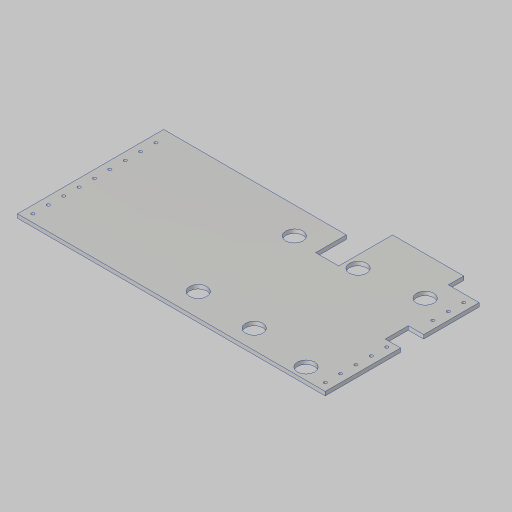
# Autodesk Inventor part: GP3-001
Saved by Autodesk Inventor 2023.5 (Build 275446000, 446)
## iProperties
Created: 2025-02-22
Part Number: GP3-001
Material: Aluminum 6061
Document SubType Name: Modeling
Designer: slick
Density: 2.7 g/cm^3
Appearance: Aluminum - Flat
Author: slick
Autodesk Inventor part; units mm, degrees
ref_plane "YZ Plane" through (0, 0, 0) normal (1, 0, 0) x (0, 1, 0)
ref_plane "XZ Plane" through (0, 0, 0) normal (0, 1, 0) x (-1, 0, 0)
ref_plane "XY Plane" through (0, 0, 0) normal (0, 0, 1) x (1, 0, 0)
sketch "Sketch1" plane through (0, 0, 0) normal (0, 1, 0) x (-1, 0, 0)
  line L0 (-254, -139.7) -> (254, -139.7)
  line L1 (254, -139.7) -> (254, 139.7)
  line L2 (254, 139.7) -> (-254, 139.7)
  line L3 (-254, 139.7) -> (-254, -139.7)
  line L4 (-254, -139.7) -> (254, 139.7) construction
  line L5 (254, -139.7) -> (-254, 139.7) construction
  point P0 (0, 0)
  dimension "d0" = 508
  dimension "d1" = 279.4
  constraints: 12 end point, 2 midpoint, 2 parallel, 1 horizontal, 1 perpendicular
  measures "d0" distance of L2.end L1.end
  measures "d1" distance of L1.end L0.end
extrude "Extrusion1" add sketch "Sketch1" along normal blind 6.35
sketch "Sketch2" plane through (0, 6.35, 0) normal (0, 1, 0) x (1, 0, 0)
  line L0 (-254, 139.7) -> (-254, -139.7) construction
  line L1 (-254, -139.7) -> (254, -139.7) construction
  line L2 (254, -139.7) -> (254, 139.7) construction
  point P0 (0, 0)
  point P1 (-241.3, -127)
  point P2 (241.3, -127)
  point P3 (-241.3, -101.6)
  point P4 (241.3, -101.6)
  point P5 (-241.3, -76.2)
  point P6 (241.3, -76.2)
  point P7 (-241.3, -50.8)
  point P8 (241.3, -50.8)
  point P9 (-241.3, -25.4)
  point P10 (241.3, -25.4)
  point P11 (-241.3, 0)
  point P12 (241.3, 0)
  point P13 (-241.3, 25.4)
  point P14 (241.3, 25.4)
  point P15 (-241.3, 50.8)
  point P16 (241.3, 50.8)
  point P17 (-241.3, 76.2)
  point P18 (241.3, 76.2)
  point P19 (-241.3, 101.6)
  point P20 (241.3, 101.6)
  point P21 (-241.3, 127)
  point P22 (241.3, 127)
  dimension "d4" = 12.7
  dimension "d5" = 12.7
  dimension "d6" = 12.7
  dimension "d9" = 25.4
  constraints: 1 horizontal alignment, 1 vertical, 20 other
  measures "d4" distance from line of point (-241.3, -127) L0
  measures "d5" distance from line of point (-241.3, -127) L1
  measures "d6" distance from line of L2 point (241.3, -127)
  measures "d9" distance of point (-241.3, -127) point (-241.3, -101.6)
hole "Hole1" at (-241.3, 6.35, 127) at (241.3, 6.35, 127) at (-241.3, 6.35, 101.6) at (241.3, 6.35, 101.6) at (-241.3, 6.35, 76.2) at (241.3, 6.35, 76.2) at (-241.3, 6.35, 50.8) at (241.3, 6.35, 50.8) at (-241.3, 6.35, 25.4) at (-241.3, 6.35, 0) at (-241.3, 6.35, -25.4) at (-241.3, 6.35, -50.8) at (241.3, 6.35, -50.8) at (241.3, 6.35, -76.2) at (241.3, 6.35, -101.6) at (241.3, 6.35, -127) at (241.3, 6.35, 25.4) at (-241.3, 6.35, -76.2) direction (0, -1, 0) diameter 5.1054 end through all clearance for "Flat Head Machine Screw (82)" size "#10" standard "Ansi Unified Screw Threads"
sketch "Sketch3" plane through (0, 6.35, 0) normal (0, 1, 0) x (1, 0, 0)
  circle A0 centre (-241.3, 50.8) radius 2.5527 construction
  circle A1 centre (-241.3, 25.4) radius 2.5527 construction
  circle A2 centre (-241.3, 0) radius 2.5527 construction
  circle A3 centre (-241.3, -25.4) radius 2.5527 construction
  circle A4 centre (-241.3, -50.8) radius 2.5527 construction
  circle A5 centre (-241.3, -76.2) radius 2.5527 construction
  circle A6 centre (-241.3, -101.6) radius 2.5527 construction
  circle A7 centre (-241.3, -127) radius 2.5527 construction
  circle A8 centre (241.3, -127) radius 2.5527 construction
  circle A9 centre (241.3, -101.6) radius 2.5527 construction
  circle A10 centre (241.3, -76.2) radius 2.5527 construction
  circle A11 centre (241.3, -50.8) radius 2.5527 construction
  circle A12 centre (241.3, 50.8) radius 2.5527 construction
  circle A13 centre (241.3, 76.2) radius 2.5527 construction
  circle A14 centre (241.3, 101.6) radius 2.5527 construction
  circle A15 centre (241.3, 127) radius 2.5527 construction
  line L0 (-254, 139.7) -> (-254, -139.7) construction
  line L1 (-254, -139.7) -> (254, -139.7) construction
  line L2 (254, -139.7) -> (254, 139.7) construction
  line L3 (254, 139.7) -> (-254, 139.7) construction
  line L4 (-254, 139.7) -> (-254, -139.7) construction
  line L5 (254, 139.7) -> (-254, 139.7) construction
  line L6 (254, 139.7) -> (203.2, 139.7)
  line L7 (203.2, 139.7) -> (203.2, 114.3)
  line L8 (203.2, 114.3) -> (254, 114.3)
  line L9 (254, 114.3) -> (254, 139.7)
  line L10 (254, 139.7) -> (-254, 139.7) construction
  line L11 (-254, 139.7) -> (47.625, 139.7)
  line L12 (47.625, 139.7) -> (47.625, 101.6)
  line L13 (47.625, 101.6) -> (-254, 101.6)
  line L14 (-254, 101.6) -> (-254, 139.7)
  line L15 (47.625, 139.7) -> (85.725, 139.7)
  line L16 (85.725, 139.7) -> (85.725, 50.8)
  line L17 (85.725, 50.8) -> (47.625, 50.8)
  line L18 (47.625, 50.8) -> (47.625, 139.7)
  line L19 (254, -139.7) -> (254, 139.7) construction
  line L20 (254, 22.86) -> (228.6, 22.86)
  line L21 (228.6, 22.86) -> (228.6, -15.24)
  line L22 (228.6, -15.24) -> (254, -15.24)
  line L23 (254, -15.24) -> (254, 22.86)
  point P0 (0, 0)
  dimension "d30" = 25.4
  dimension "d31" = 50.8
  dimension "d42" = 206.375
  dimension "d43" = 38.1
  dimension "d44" = 88.9
  dimension "d45" = 168.275
  dimension "d46" = 25.4
  dimension "d47" = 38.1
  dimension "d48" = 124.46
  constraints: 32 end point, 8 parallel, 4 horizontal, 4 perpendicular, 1 point on line
  measures "d30" distance of L6.end L7.end
  measures "d31" distance of L7.end L8.end
  measures "d42" distance between parallel lines of L2 L12
  measures "d43" distance between parallel lines of L3 L13
  measures "d44" distance of L15.end L16.end
  measures "d45" distance between parallel lines of L2 L16
  measures "d46" distance of L21.end L22.end
  measures "d47" distance between parallel lines of L22 L20
  measures "d48" distance between parallel lines of L1 L22
extrude "Extrusion2" cut sketch "Sketch3" against normal through all
sketch "Sketch4" plane through (0, 6.35, 0) normal (0, 1, 0) x (1, 0, 0)
  line L0 (-224.6258, 34.925) -> (80.1742, 34.925) construction
  line L1 (80.1742, 34.925) -> (80.1742, -79.375) construction
  line L2 (80.1742, -79.375) -> (-224.6258, -79.375) construction
  line L3 (-224.6258, -79.375) -> (-224.6258, 34.925) construction
  circle A0 centre (203.2, -120.65) radius 14.2875
  circle A1 centre (105.0189, -107.95) radius 14.2875
  circle A2 centre (203.2, 76.2) radius 14.2875
  circle A3 centre (203.2, -120.65) radius 50.8 construction
  circle A4 centre (203.2, 76.2) radius 50.8 construction
  circle A5 centre (105.0189, -107.95) radius 31.75 construction
  circle A6 centre (203.2, -120.65) radius 41.275 construction
  circle A7 centre (203.2, 76.2) radius 41.275 construction
  line L4 (254, 22.86) -> (254, 114.3) construction
  line L5 (254, 114.3) -> (203.2, 114.3) construction
  line L6 (203.2, 114.3) -> (203.2, 139.7) construction
  line L7 (203.2, 139.7) -> (85.725, 139.7) construction
  line L8 (-254, 101.6) -> (-254, -139.7) construction
  line L9 (-254, -139.7) -> (254, -139.7) construction
  circle A8 centre (-241.3, -25.4) radius 2.5527 construction
  circle A9 centre (-241.3, -50.8) radius 2.5527 construction
  circle A10 centre (-241.3, -76.2) radius 2.5527 construction
  circle A11 centre (-241.3, -101.6) radius 2.5527 construction
  circle A12 centre (-241.3, -127) radius 2.5527 construction
  circle A13 centre (241.3, -127) radius 2.5527 construction
  circle A14 centre (241.3, -101.6) radius 2.5527 construction
  circle A15 centre (241.3, -76.2) radius 2.5527 construction
  circle A16 centre (241.3, -50.8) radius 2.5527 construction
  circle A17 centre (241.3, 50.8) radius 2.5527 construction
  circle A18 centre (241.3, 76.2) radius 2.5527 construction
  circle A19 centre (241.3, 101.6) radius 2.5527 construction
  circle A20 centre (105.0189, -107.95) radius 28.575 construction
  circle A21 centre (-241.3, 50.8) radius 2.5527 projected
  line L10 (47.625, 50.8) -> (47.625, 101.6) projected
  line L11 (47.625, 101.6) -> (-254, 101.6) projected
  line L12 (85.725, 139.7) -> (85.725, 50.8) projected
  line L13 (85.725, 50.8) -> (47.625, 50.8) projected
  line L14 (254, -139.7) -> (254, -15.24) projected
  line L15 (254, -15.24) -> (228.6, -15.24) projected
  line L16 (228.6, -15.24) -> (228.6, 22.86) projected
  line L17 (228.6, 22.86) -> (254, 22.86) projected
  circle A22 centre (105.0189, 63.5) radius 14.2875
  circle A23 centre (105.0189, 63.5) radius 28.575 construction
  circle A24 centre (105.0189, 63.5) radius 31.75 construction
  circle A25 centre (6.2238, -101.6) radius 14.2875
  circle A26 centre (6.2238, 57.15) radius 14.2875
  circle A27 centre (6.2238, -101.6) radius 25.4 construction
  circle A28 centre (6.2238, -101.6) radius 22.225 construction
  circle A29 centre (6.2238, 57.15) radius 25.4 construction
  circle A30 centre (6.2238, 57.15) radius 22.225 construction
  point P0 (0, 0)
  dimension "d28" = 114.3
  dimension "d29" = 304.8
  dimension "d32" = 28.575
  dimension "d33" = 101.6
  dimension "d34" = 63.5
  dimension "d35" = 82.55
  dimension "d36" = 3.175
  dimension "d37" = 98.999
  dimension "d38" = 19.05
  dimension "d49" = 50.8
  dimension "d50" = 3.175
  dimension "d51" = 98.999
  constraints: 18 centre point, 11 equal radius, 10 coincident, 8 end point, 7 tangent, 3 vertical alignment, 2 parallel, 1 horizontal, 1 perpendicular
  measures "d28" distance of L2.end L0.start
  measures "d29" distance of L0.start L0.end
  measures "d32" diameter of A1
  measures "d33" diameter of A3
  measures "d34" diameter of A5
  measures "d35" diameter of A6
  measures "d36" radial gap between concentric circles of A5 A20
  measures "d37" distance of A0.centre A1.centre
  measures "d38" distance from line of L9 A0.centre
  measures "d49" diameter of A27
  measures "d50" radial gap between concentric circles of A27 A28
  measures "d51" distance of A1.centre A25.centre
extrude "Extrusion3" cut sketch "Sketch4" against normal blind 25.4 contours A0 | A1 | A2 | A22 | A25 | A26
equation "\"d6\" = d4"
equation "\"d51\" = d37"
body "Solid1"
